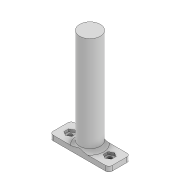
# Autodesk Inventor part: PWM3360 holder
Saved by Autodesk Inventor 2020 (Build 240168000, 168)
## iProperties
Created: 2022-03-10
Part Number: PWM3360 holder
Material: Generic
Document SubType Name: Modeling
Designer: ferrerx
Density: 1 g/cm^3
Appearance: Default
Author: ferrerx
Autodesk Inventor part; units mm, degrees
ref_plane "YZ Plane" through (0, 0, 0) normal (1, 0, 0) x (0, 1, 0)
ref_plane "XZ Plane" through (0, 0, 0) normal (0, 1, 0) x (-1, 0, 0)
ref_plane "XY Plane" through (0, 0, 0) normal (0, 0, 1) x (1, 0, 0)
sketch "Sketch1" plane through (0, 0, 0) normal (0, 1, 0) x (-1, 0, 0)
  circle A0 centre (0, 0) radius 6.3
  dimension "d0" = 12.6
  constraints: 1 centre point, 1 coincident
  measures "d0" diameter of A0
extrude "Extrusion1" add sketch "Sketch1" along normal blind 60
sketch "Sketch2" plane through (0, 0, 0) normal (0, -1, 0) x (1, 0, 0)
  line L0 (-18, 6.5) -> (18, 6.5)
  line L1 (18, 6.5) -> (18, -6.5)
  line L2 (18, -6.5) -> (-18, -6.5)
  line L3 (-18, -6.5) -> (-18, 6.5)
  line L4 (-18, 6.5) -> (18, -6.5) construction
  line L5 (18, 6.5) -> (-18, -6.5) construction
  circle A0 centre (12, 0) radius 1.35
  line L6 (0, 0) -> (0, 6.5) construction
  circle A1 centre (-12, 0) radius 1.35
  dimension "d3" = 2.7
  dimension "d4" = 12
  dimension "d5" = 36
  dimension "d6" = 13
  constraints: 14 end point, 3 midpoint, 2 centre point, 2 parallel, 1 horizontal, 1 perpendicular, 1 symmetric about line, 1 other
  measures "d3" diameter of A0
  measures "d4" distance of L6.start A0.centre
  measures "d5" distance of L1.end L2.end
  measures "d6" distance of L2.end L0.start
extrude "Extrusion2" add sketch "Sketch2" along normal blind 3
fillet "Fillet1" radius 2 1 edges at (6.3, 0, 0)
fillet "Fillet2" radius 2 4 edges at (-18, -1.5, 6.5) (-18, -1.5, -6.5) (18, -1.5, 6.5) (18, -1.5, -6.5)
sketch "Sketch3" plane through (0, 0, 0) normal (0, 1, 0) x (1, 0, 0)
  circle A0 centre (12, 0) radius 1.35 projected
  line L0 (9.5, 1.4434) -> (12, 2.8868)
  line L1 (12, 2.8868) -> (14.5, 1.4434)
  line L2 (14.5, 1.4434) -> (14.5, -1.4434)
  line L3 (14.5, -1.4434) -> (12, -2.8868)
  line L4 (12, -2.8868) -> (9.5, -1.4434)
  line L5 (9.5, -1.4434) -> (9.5, 1.4434)
  circle A1 centre (-12, 0) radius 1.35 projected
  line L6 (-14.5, 1.4434) -> (-12, 2.8868)
  line L7 (-12, 2.8868) -> (-9.5, 1.4434)
  line L8 (-9.5, 1.4434) -> (-9.5, -1.4434)
  line L9 (-9.5, -1.4434) -> (-12, -2.8868)
  line L10 (-12, -2.8868) -> (-14.5, -1.4434)
  line L11 (-14.5, -1.4434) -> (-14.5, 1.4434)
  line L12 (18, 4.5) -> (18, -4.5) projected
  line L13 (-18, -4.5) -> (-18, 4.5) projected
  point P0 (0, 0)
  dimension "d11" = 5
  dimension "d12" = 5
  constraints: 24 end point, 2 coincident, 2 parallel, 26 other
  measures "d11" distance between parallel lines of L8 L11
  measures "d12" distance between parallel lines of L2 L5
extrude "Extrusion3" cut sketch "Sketch3" against normal blind 1.5
sketch "Sketch4" plane through (0, -3, 0) normal (0, -1, 0) x (1, 0, 0)
  circle A0 centre (-8, -3.5) radius 2.5
  circle A1 centre (-8, 3.5) radius 2.5
  circle A2 centre (-12, 0) radius 1.35 projected
  line L0 (0, 0) -> (0, 6.4158) construction
  circle A3 centre (8, -3.5) radius 2.5
  circle A4 centre (8, 3.5) radius 2.5
  circle A5 centre (12, 0) radius 1.35
  dimension "d15" = 5
  dimension "d16" = 5
  dimension "d17" = 4
  dimension "d18" = 3.5
  dimension "d19" = 4
  dimension "d20" = 3.5
  constraints: 5 centre point, 3 symmetric about line, 2 end point, 1 vertical, 3 other
  measures "d15" diameter of A0
  measures "d16" diameter of A1
  measures "d17" horizontal distance of A2.centre A1.centre
  measures "d18" vertical distance of A1.centre A2.centre
  measures "d19" horizontal distance of A2.centre A0.centre
  measures "d20" vertical distance of A2.centre A0.centre
extrude "Extrusion4" cut sketch "Sketch4" against normal blind 2 contours A0 | A1 | A3 | A4
body "Solid1"
